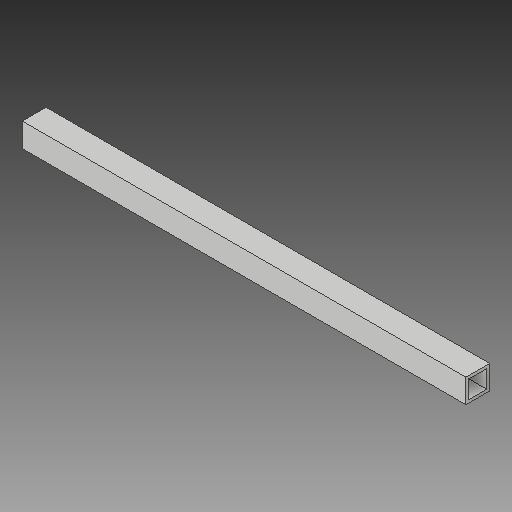
# Autodesk Inventor part: 15102898-16-P-0219
Saved by Autodesk Inventor 2017 (Build 210142000, 142)
## iProperties
Created: 2016-10-10
Part Number: 15102898-16-P-0219
Material: Generic
Document SubType Name: Modeling
Designer: gus
Density: 1 g/cm^3
Appearance: Default
Mass: 133.486 g
Surface Area: 846.502 cm^2
Volume: 133.486 cm^3
Author: gus
Autodesk Inventor part; units mm, degrees
sketch "Sketch1" plane through (0, 0, 0) normal (1, 0, 0) x (0, 1, 0)
  line L0 (0, 0) -> (25.4, 0)
  line L1 (25.4, 0) -> (25.4, -25.4)
  line L2 (0, 0) -> (0, -25.4)
  line L3 (0, -25.4) -> (25.4, -25.4)
  line L4 (22.225, -22.225) -> (22.225, -3.175)
  line L5 (22.225, -3.175) -> (3.175, -3.175)
  line L6 (3.175, -3.175) -> (3.175, -22.225)
  line L7 (3.175, -22.225) -> (22.225, -22.225)
  dimension "d1" = 25.4
  dimension "d5" = 25.4
  dimension "d7" = 25.4
  dimension "d8" = 3.175
  constraints: 16 end point, 2 perpendicular, 1 horizontal, 1 vertical, 3 other
  measures "d1" distance of L0.end L1.end
  measures "d5" distance of L0.start L0.end
  measures "d7" distance of L0.start L2.end
  measures "d8" distance between parallel lines of L1 L4
ref_plane "Work Plane1" through (121.4904, -591.0492, 62.9788) normal (-1, 0, 0) x (0, -0.0011, 1)
ref_plane "Work Plane2" through (594.413, -591.0492, 62.9788) normal (1, 0, 0) x (0, 1, 0.0011)
ref_plane "Work Plane3" through (121.4904, -685.829, -0.8415) normal (-1, 0, 0) x (0, 0, 1)
ref_plane "Work Plane4" through (572.188, -685.8218, 2.3335) normal (1, 0, 0) x (0, 1, 0)
ref_plane "Work Plane5" through (571.4614, -9.58, -1.5962) normal (1, 0, 0) x (0, 1, 0)
ref_plane "Work Plane6" through (98.5388, -9.58, -1.5962) normal (-1, 0, 0) x (0, 0, 1)
extrude "Extrusion1" add sketch "Sketch1" against normal up to surface (472.9226 mm away) from surface at 571.4614 contours L0 L1 L3 L2 | L7 L6 L5 L4
ref_plane "Work Plane7" through (98.5388, -9.554, -0.8415) normal (-1, 0, 0) x (0, 0, 1)
ref_plane "Work Plane8" through (571.4614, -9.554, -0.8415) normal (1, 0, 0) x (0, 1, 0)
extrude "Extrusion2" cut sketch "Sketch1" along normal up to surface (472.9226 mm away) from surface at 98.5388 contours L7 L6 L5 L4
body "Solid1"
